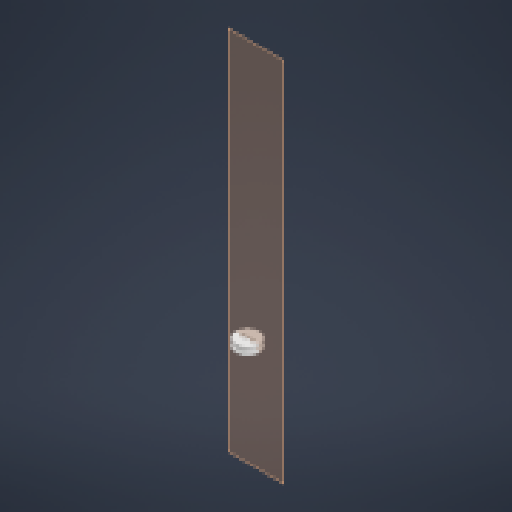
# Autodesk Inventor part: Venstre_rotator
Saved by Autodesk Inventor 2026.1 (Build 301233000, 233)
## iProperties
Created: 2025-09-28
Part Number: Venstre_rotator
Material: Generic
Document SubType Name: Modeling
Designer: Malthe Sennels
Density: 1 g/cm^3
Appearance: Default
Author: Malthe Sennels
Autodesk Inventor part; units mm, degrees
ref_plane "YZ Plane" through (0, 0, 0) normal (1, 0, 0) x (0, 1, 0)
ref_plane "XZ Plane" through (0, 0, 0) normal (0, 1, 0) x (-1, 0, 0)
ref_plane "XY Plane" through (0, 0, 0) normal (0, 0, 1) x (1, 0, 0)
ref_plane "Work Plane1" through (0, 0, 0) normal (0, 0, 1) x (1, 0, 0)
sketch "Sketch1" plane through (0, 0, 0) normal (0, 0, 1) x (1, 0, 0)
  arc A0 (13.0719, -0.4942) -> (13.1202, -0.1498) centre (10.8, 0) ccw
  circle A1 centre (10.8, 0) radius 2.325
  line L0 (10.6, -3.5) -> (10.6, -2.3164)
  line L1 (10.6, -3.5) -> (0, -3.5)
  line L2 (0, -130.1465) -> (0, 181.4158)
  line L3 (10.8, 0) -> (0, 0) construction
  line L4 (10.6, 3.5) -> (10.6, 2.3164)
  line L5 (10.6, 3.5) -> (0, 3.5)
  point P0 (0, 3.5)
  dimension "d1" = 3.5
  dimension "d12" = 4.65
  dimension "d13" = 0.2
  dimension "d14" = 10.8
  constraints: 12 end point, 4 point on circle, 4 point on line, 3 symmetric about line, 2 centre point, 1 coincident, 1 horizontal, 1 perpendicular, 1 vertical
  measures "d1" vertical distance of L0.start A0.centre
  measures "d12" diameter of A1
  measures "d13" distance from line of L0 A0.centre
  measures "d14" distance of L3.start L3.end
revolve "Revolution1" add sketch "Sketch1" angle 360 about axis through (0, -130.1465, 0) along (0, 1, 0) contours L0 L1 L2 L5 L4 A1
sketch "Sketch2" plane through (0, 3.5, 0) normal (0, 1, 0) x (1, 0, 0)
  circle A0 centre (4.5, 0) radius 2.2
  circle A1 centre (0, 0) radius 10.6 projected
  circle A2 centre (0, 0) radius 10.6 projected
  circle A3 centre (0, 0) radius 10.6 projected
  circle A4 centre (0, 0) radius 8.35
  circle A5 centre (0, 4.5) radius 2.2
  circle A6 centre (-4.5, 0) radius 2.2
  circle A7 centre (0, -4.5) radius 2.2
  point P0 (0, 0)
  dimension "d3" = 4.4
  dimension "d4" = 2.25
  dimension "d5" = 4.5
  dimension "d8" = 360
  constraints: 5 centre point, 1 coincident, 9 other
  measures "d3" diameter of A0
  measures "d4" radial gap between concentric circles of A1 A4
  measures "d5" distance of A1.centre A0.centre
extrude "Extrusion1" cut sketch "Sketch2" against normal through all contours A0 | A6
sketch "Sketch3" plane through (0, -3.5, 0) normal (0, -1, 0) x (1, 0, 0)
  line L0 (1, -1.5) -> (1.25, -1.5) projected
  line L1 (1.25, -1.5) -> (1.25, 1.5) projected
  line L2 (1.25, 1.5) -> (1, 1.5) projected
  line L3 (1, 1.5) -> (1, 3.5) projected
  line L4 (1, 3.5) -> (-1, 3.5) projected
  line L5 (-1, 3.5) -> (-1, 1.5) projected
  line L6 (-1, 1.5) -> (-1.25, 1.5) projected
  line L7 (-1.25, 1.5) -> (-1.25, -1.5) projected
  line L8 (-1.25, -1.5) -> (-1, -1.5) projected
  line L9 (-1, -1.5) -> (-1, -3.5) projected
  line L10 (-1, -3.5) -> (1, -3.5) projected
  line L11 (1, -3.5) -> (1, -1.5) projected
  circle A0 centre (4.5, 0) radius 1.55 projected
  circle A1 centre (-4.5, 0) radius 1.55 projected
  circle A2 centre (0, 0) radius 8.475 projected
  point P0 (0, 0)
extrude "Extrusion2" cut sketch "Sketch3" against normal blind 7 contours L11 L10 L9 L8 L7 L6 L5 L4 L3 L2 L1 L0
body "Solid1"
